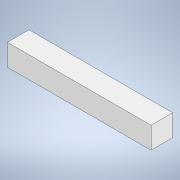
# Autodesk Inventor part: Key--Highest
Saved by Autodesk Inventor 2021 (Build 250183000, 183)
## iProperties
Created: 2021-03-17
Part Number: Key--Highest
Material: Generic
Document SubType Name: Modeling
Designer: Tom
Density: 1 g/cm^3
Appearance: White
Author: Tom
Autodesk Inventor part; units mm, degrees
ref_plane "YZ Plane" through (0, 0, 0) normal (1, 0, 0) x (0, 1, 0)
ref_plane "XZ Plane" through (0, 0, 0) normal (0, 1, 0) x (-1, 0, 0)
ref_plane "XY Plane" through (0, 0, 0) normal (0, 0, 1) x (1, 0, 0)
sketch "Sketch1" plane through (0, 0, 0) normal (0, 1, 0) x (-1, 0, 0)
  line L0 (0, 0) -> (147.6375, 0)
  line L1 (0, -22.225) -> (0, 0)
  line L2 (147.6375, 0) -> (147.6375, -22.225)
  line L3 (147.6375, -22.225) -> (0, -22.225)
  dimension "d4" = 147.6375
  dimension "d5" = 22.225
  constraints: 8 end point, 1 horizontal, 1 perpendicular, 1 vertical
  measures "d4" distance of L0.start L0.end
  measures "d5" distance of L1.start L0.start
extrude "Extrusion1" add sketch "Sketch1" against normal blind 22.225
body "Solid1"
